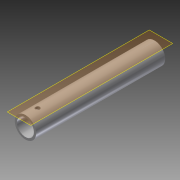
# Autodesk Inventor part: GE-13026-02
Saved by Autodesk Inventor 2013 (Build 170138000, 138)
## iProperties
Created: 2013-01-06
Part Number: GE-13026-02
Material: Steel
Document SubType Name: Modeling
Designer: Phillip
Density: 1 g/cm^3
Author: Phillip
Autodesk Inventor part; units mm, degrees
ref_plane "YZ Plane" through (0, 0, 0) normal (1, 0, 0) x (0, 1, 0)
ref_plane "XY Plane" through (0, 0, 0) normal (0, 0, 1) x (1, 0, 0)
sketch "Sketch1" plane through (0, 0, 0) normal (0, 0, 1) x (1, 0, 0)
  circle A0 centre (0, 0) radius 16.764
  circle A1 centre (0, 0) radius 13.335
  dimension "d0" = 33.528
  dimension "d2" = 26.67
  constraints: 2 centre point, 2 coincident
  measures "d0" diameter of A0
  measures "d2" diameter of A1
extrude "Extrusion1" add sketch "Sketch1" against normal blind 203.2
ref_plane "Work Plane1" through (0, 16.764, 0) normal (0, 1, 0) x (-1, 0, 0)
sketch "Sketch2" plane through (0, 16.764, 0) normal (0, 1, 0) x (-1, 0, 0)
  spline S0 degree 3 poles (0, -22.479) (-0.4316, -22.479) (-0.8912, -22.3926) (-1.7358, -22.0423) (-2.1208, -21.7786) (-2.7286, -21.1707) (-2.9923, -20.7858) (-3.3426, -19.9413) (-3.429, -19.4816) (-3.429, -19.05) (-3.429, -18.6184) (-3.3426, -18.1587) (-2.9923, -17.3142) (-2.7286, -16.9293) (-2.1208, -16.3214) (-1.7358, -16.0577) (-0.8912, -15.7074) (-0.4316, -15.621) (0, -15.621) knots 1.553636 1.553636 1.553636 1.553636 1.683104 1.683104 1.812571 1.812571 1.942043 1.942043 2.071515 2.071515 2.071515 2.200987 2.200987 2.330459 2.330459 2.459926 2.459926 2.589394 2.589394 2.589394 2.589394 projected
  spline S1 degree 3 poles (0, -22.479) (-0.4316, -22.479) (-0.8912, -22.3926) (-1.7358, -22.0423) (-2.1208, -21.7786) (-2.7286, -21.1707) (-2.9923, -20.7858) (-3.3426, -19.9413) (-3.429, -19.4816) (-3.429, -19.05) (-3.429, -18.6184) (-3.3426, -18.1587) (-2.9923, -17.3142) (-2.7286, -16.9293) (-2.1208, -16.3214) (-1.7358, -16.0577) (-0.8912, -15.7074) (-0.4316, -15.621) (0, -15.621) knots 1.553636 1.553636 1.553636 1.553636 1.683104 1.683104 1.812571 1.812571 1.942043 1.942043 2.071515 2.071515 2.071515 2.200987 2.200987 2.330459 2.330459 2.459926 2.459926 2.589394 2.589394 2.589394 2.589394 projected
  spline S2 degree 3 poles (0, -15.621) (0.4316, -15.621) (0.8912, -15.7074) (1.7358, -16.0577) (2.1208, -16.3214) (2.7286, -16.9293) (2.9923, -17.3142) (3.3426, -18.1587) (3.429, -18.6184) (3.429, -19.4816) (3.3426, -19.9413) (2.9923, -20.7858) (2.7286, -21.1707) (2.1208, -21.7786) (1.7358, -22.0423) (0.8912, -22.3926) (0.4316, -22.479) (0, -22.479) knots 0.517879 0.517879 0.517879 0.517879 0.647346 0.647346 0.776813 0.776813 0.906285 0.906285 1.035757 1.035757 1.16523 1.16523 1.294702 1.294702 1.424169 1.424169 1.553636 1.553636 1.553636 1.553636 projected
  point P0 (0, 0)
extrude "Extrusion2" cut sketch "Sketch2" against normal through all
body "Solid1"
